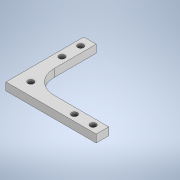
# Autodesk Inventor part: Step-back spacer -electronics enc
Saved by Autodesk Inventor 2021 (Build 250183000, 183)
## iProperties
Created: 2020-09-03
Part Number: Step-back spacer -electronics enc
Material: Generic
Document SubType Name: Modeling
Designer: jgray
Density: 1 g/cm^3
Appearance: Default
Author: jgray
Autodesk Inventor part; units mm, degrees
ref_plane "YZ Plane" through (0, 0, 0) normal (1, 0, 0) x (0, 1, 0)
ref_plane "XZ Plane" through (0, 0, 0) normal (0, 1, 0) x (-1, 0, 0)
ref_plane "XY Plane" through (0, 0, 0) normal (0, 0, 1) x (1, 0, 0)
sketch "Sketch1" plane through (0, 0, 0) normal (0, 1, 0) x (-1, 0, 0)
  line L0 (0, 0) -> (58, 0)
  line L1 (58, 0) -> (58, -50)
  line L2 (58, -50) -> (0, -50)
  line L3 (0, -50) -> (0, 0)
  line L4 (0, -50) -> (50, -50)
  line L5 (50, -50) -> (50, -23)
  line L6 (35, -8) -> (0, -8)
  line L7 (0, -8) -> (0, -50)
  arc A0 (50, -23) -> (35, -8) centre (35, -23) ccw
  line L8 (54, -53.5159) -> (54, 28.6039) construction
  line L9 (-7.6056, -4) -> (76.8297, -4) construction
  point P0 (50, -8)
  point P1 (6, -4)
  point P2 (18, -4)
  point P3 (54, -32)
  point P4 (54, -44)
  point P5 (50, -8)
  dimension "d0" = 58
  dimension "d1" = 50
  dimension "d2" = 50
  dimension "d3" = 42
  dimension "d4" = 15
  dimension "d5" = 6
  dimension "d6" = 18
  dimension "d7" = 18
  dimension "d8" = 6
  constraints: 20 end point, 6 point on line, 4 parallel, 3 horizontal, 2 perpendicular, 2 point on circle, 2 tangent, 1 centre point, 1 coincident, 1 vertical, 2 other
  measures "d0" distance of L1.end L2.end
  measures "d1" distance of L0.end L1.end
  measures "d2" distance of L6.end point (50, -8)
  measures "d3" distance of point (50, -8) L4.end
  measures "d4" radius of A0
  measures "d5" distance from line of L2 point (54, -44)
  measures "d6" distance from line of point (54, -32) L2
  measures "d7" distance from line of L3 point (18, -4)
  measures "d8" distance from line of L3 point (6, -4)
extrude "Extrusion1" add sketch "Sketch1" against normal blind 5 contours L0 L1 L2 L5 A0 L6 L3
hole "Hole1" at (-6, 0, -4) at (-18, 0, -4) at (-54, 0, -32) at (-54, 0, -44) at (-50, 0, -8) direction (0, -1, 0) diameter 3.8 end through all
body "Solid1"
